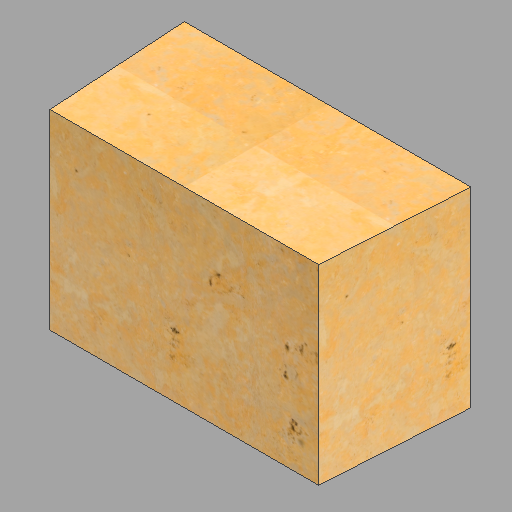
# Autodesk Inventor part: F1
Saved by Autodesk Inventor 2023 (Build 270158030, 158C)
## iProperties
RuleStatus: InUse
Created: 2022-05-23
Part Number: F1
Material: Granite, Cut, Polished
Document SubType Name: Modeling
Designer: awelt
Mass: 666544 g
Surface Area: 24483.6 cm^2
Volume: 246868 cm^3
Density: 2.7 g/cm^3
Appearance: Amber Select
AfterDocSave0: Convert in3 volume to ft3
in3 to ft3: 0.01
TEST: 0.005
Author: awelt
Autodesk Inventor part; units mm, degrees
ref_plane "YZ Plane" through (0, 0, 0) normal (1, 0, 0) x (0, 1, 0)
ref_plane "XZ Plane" through (0, 0, 0) normal (0, 1, 0) x (-1, 0, 0)
ref_plane "XY Plane" through (0, 0, 0) normal (0, 0, 1) x (1, 0, 0)
sketch "Sketch1" plane through (0, 0, 0) normal (0, 1, 0) x (-1, 0, 0)
  line L0 (0, 0) -> (-914.4, 0)
  line L1 (-28.6444, 457.2) -> (-885.7556, 457.2)
  line L2 (0, 0) -> (-28.6444, 457.2)
  line L3 (-914.4, 0) -> (-885.7556, 457.2)
  line L4 (-457.2, 0) -> (-457.2, 457.2) construction
  dimension "d0" = 914.4
  dimension "d2" = 457.2
  dimension "d3" = 7.17
  constraints: 10 end point, 2 horizontal, 2 midpoint, 1 other
  measures "d0" distance of L0.start L0.end
  measures "d2" distance between parallel lines of L0 L1
  measures "d3" angle of L3 L2
extrude "Extrusion1" add sketch "Sketch1" along normal blind 609.6
body "Solid1"
